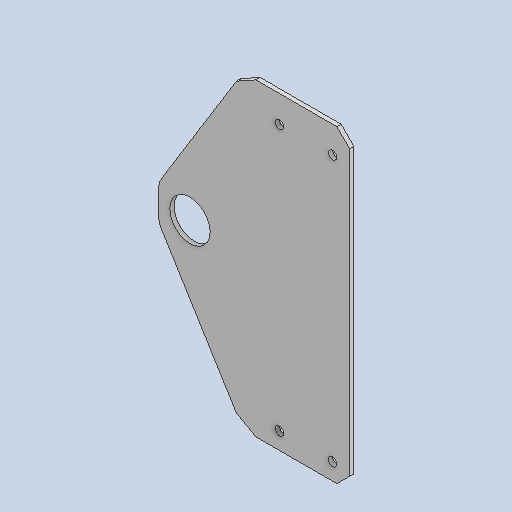
# Autodesk Inventor part: Piston_A_beam_hinge
Saved by Autodesk Inventor 2025.2 (Build 292293000, 293)
## iProperties
Created: 2025-04-29
Part Number: Piston_A_beam_hinge
Material: Generic
Document SubType Name: Sheet Metal
Designer: Caspe
Density: 1 g/cm^3
Sheet Metal Rule: Default_mm
Appearance: Default
Author: Caspe
Autodesk Inventor part; units mm, degrees
ref_plane "YZ Plane" through (0, 0, 0) normal (1, 0, 0) x (0, 1, 0)
ref_plane "XZ Plane" through (0, 0, 0) normal (0, 1, 0) x (-1, 0, 0)
ref_plane "XY Plane" through (0, 0, 0) normal (0, 0, 1) x (1, 0, 0)
sketch "Sketch1" plane through (0, 0, 0) normal (0, 0, 1) x (1, 0, 0)
  circle A0 centre (0, 0) radius 2
  circle A1 centre (25, 0) radius 2
  line L0 (0, 0) -> (0, 2)
  circle A2 centre (0, 125) radius 2
  circle A3 centre (25, 125) radius 2
  line L1 (33, -8) -> (-57.1446, -8)
  line L2 (-57.1446, -8) -> (-57.1446, 137.5528)
  line L3 (-57.1446, 137.5528) -> (33, 137.5528)
  line L4 (33, 137.5528) -> (33, -8)
  line L5 (-57.1446, 64.7764) -> (33, 64.7764)
  circle A4 centre (-42.1446, 64.7764) radius 9.5
  point P0 (0, 127)
  dimension "d0" = 4
  dimension "d1" = 4
  dimension "d2" = 25
  dimension "d5" = 125
  dimension "d10" = 8
  dimension "d11" = 8
  dimension "d12" = 12.5528
  dimension "d13" = 19
  dimension "d14" = 15
  measures "d1" diameter of A1
  measures "d2" distance of A1.centre L0.start
  measures "d5" distance of L0.start point (0, 125)
  measures "d10" distance from line of L0.start L1
  measures "d11" distance from line of L4 A1.centre
  measures "d12" distance from line of A3.centre L3
  measures "d13" diameter of A4
  measures "d14" distance from line of L2 A4.centre
extrude "Plate1" add sketch "Sketch1" along normal blind 2 contours L1 L2 L5 A4 L4 | L5 A4 L2 L3 L4
chamfer "Corner Chamfer1" distance 40 distance2 65 1 edges at (-57.1446, 137.5528, 1) measured on face at (-56.6446, 137.5528, 1)
chamfer "Corner Chamfer2" distance 40 distance2 65 1 edges at (-57.1446, -8, 1) measured on face at (-56.6446, -8, 1)
fillet "Corner Round1" radius 12 2 edges at (-57.1446, 72.5528, 1) (-57.1446, 57, 1)
chamfer "Corner Chamfer3" distance 6 angle 45 4 edges at (33, 137.5528, 1) (-17.1446, 137.5528, 1) (-17.1446, -8, 1) (33, -8, 1)
equation "\"d0\" = rivet_diameter"
equation "\"d1\" = rivet_diameter"
equation "\"d15\" = Thickness"
equation "\"d5\" = 0.5 * rivet_displacement"
equation "\"Thickness\" = plate_thickness"
equation "\"BendRadius\" = Thickness"
equation "\"BendReliefWidth\" = Thickness"
equation "\"BendReliefDepth\" = 0.5 * Thickness"
equation "\"CornerReliefSize\" = 4 * Thickness"
equation "\"MinimumRemnant\" = 2 * Thickness"
equation "\"TransitionRadius\" = BendRadius"
equation "\"JacobiRadiusSize\" = BendRadius"
equation "\"GapSize\" = Thickness"
equation "\"A_B_spacing\" = 2"
equation "\"A_joint_tolerance\" = 3"
equation "\"l___________\" = 0"
equation "\"l__________\" = 0"
equation "\"l_________\" = 0"
equation "\"rivet_diameter\" = 4"
equation "\"plate_thickness\" = 2"
equation "\"l________\" = 0"
equation "\"L_Piston_Top\" = 25"
equation "\"L_Piston_Bottom\" = 21"
equation "\"rivet_displacement\" = 250"
body "Solid1"
